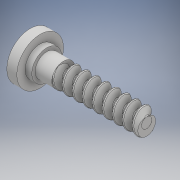
# Autodesk Inventor part: coffee_screw
Saved by Autodesk Inventor 2017 (Build 210142000, 142)
## iProperties
Part Number: coffee_screw
Material: Типовые
Document SubType Name: Modeling
Designer: Tolya
Density: 1 g/cm^3
Appearance: По умолчанию
Author: Tolya
Autodesk Inventor part; units mm, degrees
ref_plane "YZ Plane" through (0, 0, 0) normal (1, 0, 0) x (0, 1, 0)
ref_plane "XZ Plane" through (0, 0, 0) normal (0, 1, 0) x (-1, 0, 0)
ref_plane "XY Plane" through (0, 0, 0) normal (0, 0, 1) x (1, 0, 0)
sketch "Эскиз1" plane through (0, 0, 0) normal (0, 0, 1) x (1, 0, 0)
  line L0 (0, 0) -> (30, 0)
  line L1 (30, 0) -> (30, 3.5)
  line L2 (30, 3.5) -> (0, 3.5)
  line L3 (0, 3.5) -> (0, 0)
  line L4 (0, 3.5) -> (0, 4.5)
  line L5 (0, 4.5) -> (-2, 4.5)
  line L6 (-2, 4.5) -> (-2, 0)
  line L7 (-2, 0) -> (0, 0)
  line L8 (-2, 4.5) -> (-2, 7)
  line L9 (-2, 7) -> (-5, 7)
  line L10 (-5, 7) -> (-5, 0)
  line L11 (-5, 0) -> (0, 0)
  dimension "d0" = 30
  dimension "d1" = 3.5
  dimension "d2" = 1
  dimension "d3" = 2
  dimension "d4" = 2.5
  dimension "d5" = 3
  constraints: 24 end point, 8 perpendicular, 2 vertical, 1 collinear, 1 horizontal
  measures "d0" distance of L0.start L0.end
  measures "d1" distance of L0.end L1.end
  measures "d2" distance of L2.end L4.end
  measures "d3" distance of L4.end L5.end
  measures "d4" distance of L5.end L8.end
  measures "d5" distance of L8.end L9.end
revolve "Вращение1" add sketch "Эскиз1" angle 360 about axis through (0, 0, 0) along (1, 0, 0)
thread "Резьба1" size "7x3.2" class "h15" standard "DIN Wood Screw Thread" length 25.006
sketch "Эскиз3" plane through (30, 0, 0) normal (0, -1, 0) x (0, 0, 1)
  line L0 (3.5, 0) -> (3.5, 25.006)
  line L1 (3.5, 25.006) -> (1.5423, 25.006)
  line L2 (1.5423, 25.006) -> (1.5423, 0)
  line L3 (1.5423, 0) -> (3.5, 0)
  line L4 (0, -10.9586) -> (0, 42.6598) projected
  constraints: 8 end point
revolve "Вращение2" cut sketch "Эскиз3" angle 360 about axis through (30, 0, 0) along (-1, 0, 0)
sketch "Эскиз4" plane through (30, 0, 0) normal (0, -1, 0) x (0, 0, 1)
  line L0 (3.5, 0) -> (3.5, 25.006)
  line L1 (3.5, 25.006) -> (1.5423, 25.006)
  line L2 (1.5423, 25.006) -> (1.5423, 0)
  line L3 (1.5423, 0) -> (3.5, 0)
  line L4 (0, -10.9586) -> (0, 42.6598) projected
  constraints: 8 end point
revolve "Вращение3" add sketch "Эскиз4" angle 360 about axis through (30, 0, 0) along (-1, 0, 0) separate body
sketch "Эскиз2" plane through (30, 0, 0) normal (0, 1, 0) x (-1, 0, 0)
  line L0 (-1.7774, -1.7025) -> (-1.5001, -1.7025) construction
  line L1 (0.2772, -3.3401) -> (-0.0001, -3.8203) construction
  line L2 (-3.0001, -3.8203) -> (-3.2774, -3.3401) construction
  line L3 (-1.2228, -1.7025) -> (-1.5001, -1.2223) construction
  line L4 (-1.5001, -1.2223) -> (-1.7774, -1.7025) construction
  line L5 (-3.0001, -3.8203) -> (-2.7228, -3.3401) construction
  line L6 (-1.2228, -1.7025) -> (-0.2774, -3.3401)
  line L7 (-3.2774, -3.3401) -> (-2.7228, -3.3401) construction
  arc A0 (-3.2774, -3.3401) -> (-3.0001, -3.5002) centre (-3.0001, -3.18) ccw construction
  line L8 (0.2772, -3.3401) -> (-0.2774, -3.3401) construction
  line L9 (-3.0001, -3.8203) -> (-3.0001, -3.3401) construction
  line L10 (-0.0001, -3.8203) -> (-0.0001, -3.3401) construction
  line L11 (-1.5001, -1.2223) -> (-1.5001, -1.5424) construction
  line L12 (-3.0001, -3.5002) -> (-0.0001, -3.5002)
  arc A1 (-3.0001, -3.5002) -> (-2.7228, -3.3401) centre (-3.0001, -3.18) ccw
  line L13 (-0.2774, -3.3401) -> (-0.0001, -3.8203) construction
  line L14 (-2.7228, -3.3401) -> (-1.7774, -1.7025)
  line L15 (-0.0001, -0.0002) -> (-0.0001, 0.0177)
  line L16 (-0.0001, 0.0177) -> (-0.0001, -0.0002)
  line L17 (-0.0001, -0.0002) -> (0.0334, -0.0002)
  arc A2 (-0.2774, -3.3401) -> (-0.0001, -3.5002) centre (-0.0001, -3.18) ccw
  arc A3 (-0.0001, -3.5002) -> (0.2772, -3.3401) centre (-0.0001, -3.18) ccw construction
  arc A4 (-1.5001, -1.5424) -> (-1.7774, -1.7025) centre (-1.5001, -1.8626) ccw
  arc A5 (-1.2228, -1.7025) -> (-1.5001, -1.5424) centre (-1.5001, -1.8626) ccw
  line L18 (-1.5001, -1.5424) -> (-1.5001, -1.7025) construction
  line L19 (-1.5001, -1.7025) -> (-1.2228, -1.7025) construction
  dimension "d9" = 60
  dimension "d10" = 0.4803
  dimension "d11" = 0.4803
  dimension "Эскиз2_ThreadOffset" = 0
  dimension "Эскиз2_MajorRadius" = 3.5
  dimension "d14" = 3
  dimension "Эскиз2_MinorRadius" = 1.5423
  constraints: 40 end point, 12 point on circle, 10 parallel, 8 tangent, 6 centre point, 6 collinear, 2 midpoint, 2 point on line, 1 horizontal, 1 perpendicular, 3 other
  measures "d9" angle of L6 L14
  measures "d10" distance of L3.end L0.end
  measures "d11" distance of L1.end L10.end
  measures "Эскиз2_ThreadOffset" distance between parallel lines of L15 L10
  measures "Эскиз2_MajorRadius" distance from line of L12 L15.start
  measures "d14" distance from line of L1.end L9
  measures "Эскиз2_MinorRadius" distance edge to line of A5 L17
coil "Пружина1" sketch "Эскиз2" operation cut axis through (30, 0, 0) along (-1, 0, 0) pitch 3.003 turns 10.325008 hand right bodies 2
equation "\"d9\" = d16"
equation "\"d10\" = 0.160083 * Эскиз2_Pitch"
equation "\"d11\" = 0.160083 * Эскиз2_Pitch"
equation "\"d14\" = Эскиз2_Pitch"
equation "\"d16\" = 60deg"
equation "\"Эскиз2_Pitch\" = 3"
